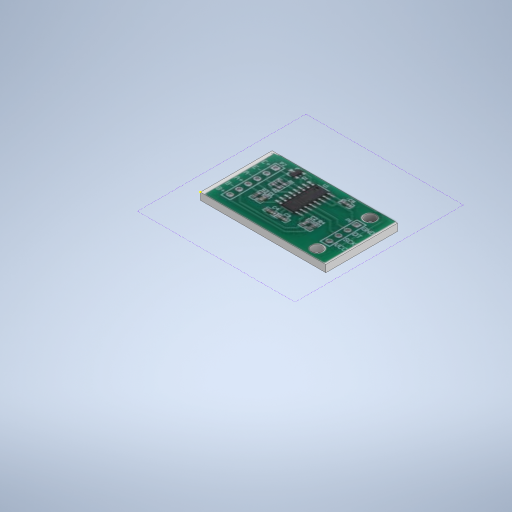
# Autodesk Inventor part: hx711
Saved by Autodesk Inventor 2024.3 (Build 283343000, 343)
## iProperties
Created: 2025-01-01
Part Number: hx711
Material: Generic
Document SubType Name: Modeling
Designer: email
Density: 1 g/cm^3
Appearance: Default
Author: email
Autodesk Inventor part; units mm, degrees
ref_plane "YZ Plane" through (0, 0, 0) normal (1, 0, 0) x (0, 1, 0)
ref_plane "XZ Plane" through (0, 0, 0) normal (0, 1, 0) x (-1, 0, 0)
ref_plane "XY Plane" through (0, 0, 0) normal (0, 0, 1) x (1, 0, 0)
sketch "Sketch1" plane through (0, 0, 0) normal (0, 1, 0) x (-1, 0, 0)
  line L0 (4.0913, -33.3854) -> (-39.8699, -33.3854) construction
  line L1 (-39.8699, -33.3854) -> (-39.8699, 13.6146) construction
  line L2 (-39.8699, 13.6146) -> (4.0913, 13.6146) construction
  line L3 (4.0913, 13.6146) -> (4.0913, -33.3854) construction
  line L4 (0, 0) -> (-35, 0)
  line L5 (-35, 0) -> (-35, -20)
  line L6 (-35, -20) -> (0, -20)
  line L7 (0, -20) -> (0, 0)
  circle A0 centre (-29.92, -17.46) radius 1.5
  circle A1 centre (-29.92, -2.54) radius 1.5
  dimension "d1" = 20
  dimension "d6" = 35
  dimension "d17" = 47
  dimension "d22" = 3
  dimension "d23" = 3
  dimension "d24" = 5.08
  dimension "d25" = 5.08
  dimension "d26" = 2.54
  dimension "d27" = 2.54
  constraints: 8 end point, 2 centre point, 2 parallel, 1 horizontal, 1 perpendicular, 2 other
  measures "d1" distance of L4.end L5.end
  measures "d6" distance of L5.end L6.end
  measures "d17" distance of L0.end L1.end
  measures "d22" diameter of A0
  measures "d23" diameter of A1
  measures "d24" distance from line of L5 A0.centre
  measures "d25" distance from line of L5 A1.centre
  measures "d26" distance from line of L6 A0.centre
  measures "d27" distance from line of L4 A1.centre
extrude "Extrusion1" add sketch "Sketch1" along normal blind 2
sketch "Sketch2" plane through (0, 2, 0) normal (0, 1, 0) x (1, 0, 0)
  line L0 (-4.1581, 33.5847) -> (39.8031, 33.5847) construction
  line L1 (39.8031, 33.5847) -> (39.8031, -13.4153) construction
  line L2 (39.8031, -13.4153) -> (-4.1581, -13.4153) construction
  line L3 (-4.1581, -13.4153) -> (-4.1581, 33.5847) construction
  point P0 (0, 0)
  dimension "d33" = 47
  constraints: 2 other
  measures "d33" distance of L0.end L1.end
body "Solid1"
